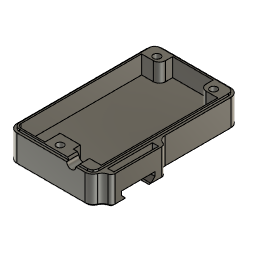
DisplayCaseBottom (Autodesk Fusion 360 design; units mm, degrees)
Autodesk Fusion 360 part; units mm, degrees
sketch "Skizze1" plane through (0, 0, 0) normal (0, 0, 1) x (1, 0, 0)
  line L0 (0, 0) -> (20.8, 0)
  line L1 (20.8, 0) -> (20.8, 72)
  line L2 (20.8, 72) -> (0, 72)
  line L3 (0, 72) -> (0, 0)
  dimension "d1" = 20.8
  dimension "d2" = 72
  constraint horizontal L0
  constraint vertical L1
  constraint horizontal L2
  constraint vertical L3
  constraint coincident L0.start L3.end
  measures "d1" distance of L0.start L0.end
  measures "d2" distance of L0.end L1.end
extrude "Extrusion1" add sketch "Skizze1" along normal blind 6
sketch "Skizze2" plane through (0, 0, 0) normal (-1, 0, 0) x (0, -1, 0)
  line L0 (-72, 0) -> (0, 0)
  line L1 (0, 0) -> (0, 6)
  line L2 (0, 6) -> (-72, 6)
  line L3 (-72, 6) -> (-72, 0)
  line L4 (-24.5, 0) -> (-12, 0)
  line L5 (-12, 0) -> (-12, 1)
  line L6 (-12, 1) -> (-10, 3)
  line L7 (-10, 3) -> (-10, 5)
  line L8 (-10, 5) -> (-26.5, 5)
  line L9 (-26.5, 5) -> (-26.5, 3)
  line L10 (-26.5, 3) -> (-24.5, 1)
  line L11 (-24.5, 1) -> (-24.5, 0)
  dimension "d5" = 16.5
  dimension "d6" = 1
  dimension "d7" = 1
  dimension "d8" = 45
  dimension "d9" = 45
  dimension "d10" = 2
  dimension "d11" = 2
  dimension "d12" = 2
  dimension "d13" = 10
  constraint coincident L0 L4.start
  constraint coincident L0 L4.end
  constraint perpendicular L4 L5
  constraint perpendicular L4 L7
  constraint perpendicular L7 L8
  constraint perpendicular L8 L9
  constraint perpendicular L8 L11
  measures "d5" distance of L7.end L8.end
  measures "d6" distance of L4.start L10.end
  measures "d7" distance of L4.end L5.end
  measures "d8" angle of L5 L6
  measures "d9" angle of L10 L11
  measures "d10" vertical distance of L5.end L6.end
  measures "d11" distance of L6.end L7.end
  measures "d12" distance of L8.end L9.end
  measures "d13" horizontal distance of L0.end L7.end
extrude "Extrusion2" cut sketch "Skizze2" against normal through all contours L0 L4 L5 L6 L7 L8 L9 L10 L11
sketch "Skizze3" plane through (0, 0, 6) normal (0, 0, 1) x (-1, 0, 0)
  line L0 (0, -72) -> (0, 0)
  line L1 (0, 0) -> (-20.8, 0)
  line L2 (-20.8, 0) -> (-20.8, -72)
  line L3 (-20.8, -72) -> (0, -72)
  line L4 (0, -72) -> (-20.8, -72)
  line L5 (-20.8, -72) -> (-20.8, 0)
  line L6 (-20.8, 0) -> (0, 0)
  line L7 (0, 0) -> (0, -2)
  line L8 (0, -2) -> (-18.8, -2)
  line L9 (-18.8, -2) -> (-18.8, -70)
  line L10 (-18.8, -70) -> (0, -70)
  line L11 (0, -70) -> (0, -72)
  dimension "d15" = 2
  dimension "d16" = 2
  dimension "d17" = 2
  constraint coincident L0.start L3.end
  constraint coincident L2.end L3.start
  constraint coincident L1.end L2.start
  constraint coincident L0.end L1.start
  constraint coincident L0 L7.end
  constraint perpendicular L7 L8
  constraint perpendicular L8 L9
  constraint coincident L0 L10.end
  constraint perpendicular L0 L10
  measures "d15" distance of L0.start L10.end
  measures "d16" distance of L5 L9
  measures "d17" distance of L6 L8
extrude "Extrusion3" add sketch "Skizze3" along normal blind 8 contours L0 L1 L2 L3 L4 L5 L6 L7 L8 L9 L10 L11
sketch "Skizze4" plane through (0, 0, 14) normal (0, 0, 1) x (-1, 0, 0)
  line L0 (0, -70) -> (-18.8, -70)
  line L1 (-18.8, -70) -> (-18.8, -2)
  line L2 (-18.8, -2) -> (0, -2)
  line L3 (0, -70) -> (-18.8, -70)
  line L4 (-18.8, -70) -> (-18.8, -2)
  line L5 (-18.8, -2) -> (0, -2)
  line L6 (0, -2) -> (0, -1.2)
  line L7 (0, -1.2) -> (-19.6, -1.2)
  line L8 (-19.6, -1.2) -> (-19.6, -70.8)
  line L9 (-19.6, -70.8) -> (0, -70.8)
  line L10 (0, -70.8) -> (0, -70)
  dimension "d49" = 0.8
  dimension "d50" = 0.8
  dimension "d51" = 0.8
  constraint coincident L0.start L3.start
  constraint coincident L0.end L1.start
  constraint coincident L1.end L2.start
  constraint coincident L2.end L5.end
  constraint perpendicular L2 L6
  constraint perpendicular L6 L7
  constraint perpendicular L3 L8
  constraint perpendicular L8 L9
  constraint perpendicular L3 L10
  measures "d49" distance of L9.end L0.start
  measures "d50" distance of L0.end L8
  measures "d51" distance of L2.end L6.end
extrude "Extrusion4" add sketch "Skizze4" along normal blind 1
sketch "Skizze5" plane through (0, 0, 6) normal (0, 0, 1) x (-1, 0, 0)
  line L0 (0, -2) -> (-18.8, -2)
  line L1 (-18.8, -2) -> (-18.8, -70)
  line L2 (-18.8, -70) -> (0, -70)
  line L3 (0, -70) -> (0, -2)
  line L4 (-18.8, -70) -> (-10, -70)
  line L5 (-10, -70) -> (-10, -63.5)
  line L6 (-10, -63.5) -> (-18.8, -63.5)
  line L7 (-18.8, -63.5) -> (-18.8, -70)
  dimension "d25" = 10
  dimension "d26" = 6.5
  constraint horizontal L4
  constraint vertical L5
  constraint horizontal L6
  constraint vertical L7
  constraint coincident L1.end L2.start
  measures "d25" distance of L3 L5.end
  measures "d26" distance of L4.end L5.end
extrude "Extrusion5" add sketch "Skizze5" along normal blind 9 contours L1 L2 L4 L5 L6 L7
sketch "Skizze7" plane through (0, 0, 0) normal (0, 0, -1) x (1, 0, 0)
  line L0 (20.8, -24.5) -> (0, -24.5)
  line L1 (0, -24.5) -> (0, -72)
  line L2 (0, -72) -> (20.8, -72)
  line L3 (20.8, -72) -> (20.8, -24.5)
  point P0 (14, -66.25)
  dimension "d31" = 14
  dimension "d32" = 5.75
  measures "d31" horizontal distance of origin P0
  measures "d32" distance of L2 P0
hole "Bohrung1" at (14, 66.25, 0) direction (0, 0, 1) diameter 3.5 end through all counterbore diameter 6.5 counterbore depth 4
chamfer "Fase1" distance 1.5 angle 45 1 edges at (15.6316, 66.8828, 4)
sketch "Skizze8" plane through (0, 0, 6) normal (0, 0, 1) x (-1, 0, 0)
  line L0 (-18.8, -63.5) -> (-10, -63.5)
  line L1 (-10, -63.5) -> (-10, -70)
  line L2 (-10, -70) -> (0, -70)
  line L3 (0, -70) -> (0, -2)
  line L4 (0, -2) -> (-18.8, -2)
  line L5 (-18.8, -2) -> (-18.8, -63.5)
  line L6 (0, -2) -> (-5, -2)
  line L7 (-5, -2) -> (-5, -9.5)
  line L8 (-5, -9.5) -> (0, -9.5)
  line L9 (0, -9.5) -> (0, -2)
  dimension "d38" = 5
  dimension "d39" = 9.5
  constraint horizontal L6
  constraint vertical L7
  constraint horizontal L8
  constraint vertical L9
  constraint coincident L3.end L4.start
  measures "d38" distance of L3.end L6.end
  measures "d39" vertical distance of origin L7.end
extrude "Extrusion6" add sketch "Skizze8" along normal blind 9 contours L3 L4 L6 L7 L8 L9
sketch "Skizze9" plane through (0, 0, 0) normal (0, 0, -1) x (1, 0, 0)
  line L0 (0, -12) -> (20.8, -12)
  line L1 (20.8, -12) -> (20.8, 0)
  line L2 (20.8, 0) -> (0, 0)
  line L3 (0, 0) -> (0, -12)
  point P0 (0, -4.5)
  dimension "d42" = 4.5
  constraint coincident L3 P0
  measures "d42" distance of L2.end P0
hole "Bohrung2" at (0, 4.5, 0) direction (0, 0, 1) diameter 3.5 depth 16 tip angle 180 counterbore diameter 6.5 counterbore depth 6
chamfer "Fase2" distance 1.5 angle 45 1 edges at (1.75, 4.5, 6)
fillet "Abrundung6" radius 2 1 edges at (18.8, 2, 10.5)
fillet "Abrundung2" radius 2.8 2 edges at (19.6, 1.2, 14.5) (19.6, 70.8, 14.5)
fillet "Abrundung4" radius 4 2 edges at (20.8, 0, 7) (20.8, 72, 7)
fillet "Abrundung5" radius 3 1 edges at (10, 63.5, 10.5)
mirror "Spiegeln1" about plane through (0, 0, 0) normal (1, 0, 0) of bodies 1 merged
sketch "Skizze11" plane through (0, 0, 6) normal (0, 0, 1) x (-1, 0, 0)
  line L0 (-18.8, -4) -> (-18.8, -63.5)
  line L1 (-18.8, -63.5) -> (-13, -63.5)
  arc A0 (-10, -66.5) -> (-13, -63.5) centre (-13, -66.5) ccw
  line L2 (-10, -66.5) -> (-10, -70)
  line L3 (-10, -70) -> (10, -70)
  line L4 (10, -70) -> (10, -66.5)
  arc A1 (13, -63.5) -> (10, -66.5) centre (13, -66.5) ccw
  line L5 (13, -63.5) -> (18.8, -63.5)
  line L6 (18.8, -63.5) -> (18.8, -4)
  line L7 (16.8, -2) -> (5, -2)
  line L8 (5, -2) -> (5, -9.5)
  line L9 (5, -9.5) -> (-5, -9.5)
  line L10 (-5, -9.5) -> (-5, -2)
  line L11 (-5, -2) -> (-16.8, -2)
  line L12 (-5, -2) -> (-18.8, -2)
  line L13 (-18.8, -2) -> (-18.8, -6)
  line L14 (-18.8, -6) -> (-5, -6)
  line L15 (-5, -6) -> (-5, -2)
  arc A2 (-16.8, -2) -> (-18.8, -4) centre (-16.8, -4) ccw
  arc A3 (18.8, -4) -> (16.8, -2) centre (16.8, -4) ccw
  dimension "d68" = 4
  constraint horizontal L12
  constraint vertical L13
  constraint horizontal L14
  constraint vertical L15
  constraint coincident L0 L13.end
  constraint coincident L10.end L11.start
  measures "d68" distance of L12.end L13.end
extrude "Extrusion7" add sketch "Skizze11" along normal blind 9 contours L0 L10 L11 L12 L13 L14 L15 A2 | L12 L13 A2
sketch "Skizze10" plane through (0, 0, 0) normal (0, -1, 0) x (1, 0, 0)
  line L0 (16.8, 0) -> (16.8, 14)
  line L1 (16.8, 14) -> (-16.8, 14)
  line L2 (-16.8, 14) -> (-16.8, 0)
  circle A0 centre (10, 14) radius 2.25
  line L3 (-16.8, 0) -> (16.8, 0)
  dimension "d66" = 4.5
  dimension "d67" = 10
  constraint coincident L1 A0.centre
  measures "d66" diameter of A0
  measures "d67" horizontal distance of origin A0.centre
extrude "Extrusion8" cut sketch "Skizze10" against normal blind 12 contours L1 A0 | L1 A0
chamfer "Fase5" distance 1 angle 45 3 edges at (7.9844, 3.6, 15) (12.0156, 3.6, 15) (7.9844, 3.6, 15)
sketch "Skizze16" plane through (20.8, 0, 0) normal (1, 0, 0) x (0, 1, 0)
  line L0 (68, 0) -> (68, 14)
  line L1 (68, 14) -> (4, 14)
  line L2 (4, 14) -> (4, 0)
  line L3 (4, 0) -> (12, 0)
  line L4 (12, 0) -> (12, 1)
  line L5 (12, 1) -> (10, 3)
  line L6 (10, 3) -> (10, 5)
  line L7 (10, 5) -> (26.5, 5)
  line L8 (26.5, 5) -> (26.5, 3)
  line L9 (26.5, 3) -> (24.5, 1)
  line L10 (24.5, 1) -> (24.5, 0)
  line L11 (24.5, 0) -> (68, 0)
  line L12 (5, 14) -> (31.5, 14)
  line L13 (31.5, 14) -> (31.5, 0)
  line L14 (31.5, 0) -> (5, 0)
  line L15 (5, 0) -> (5, 14)
  dimension "d100" = 5
  dimension "d101" = 5
  constraint horizontal L12
  constraint vertical L13
  constraint horizontal L14
  constraint vertical L15
  constraint coincident L11 L13.end
  constraint coincident L1 L12.start
  measures "d100" horizontal distance of L7.end L13.end
  measures "d101" distance of L6.end L15
extrude "Extrusion12" add sketch "Skizze16" along normal blind 4 contours L1 L3 L4 L5 L6 L7 L8 L9 L10 L11 L12 L13 L14 L15
sketch "Skizze17" plane through (0, 0, 14) normal (0, 0, 1) x (-1, 0, 0)
  line L0 (-12.25, -1.2) -> (-12.25, 0)
  line L1 (-12.25, 0) -> (-16.8, 0)
  arc A0 (-16.8, 0) -> (-20.8, -4) centre (-16.8, -4) ccw
  line L2 (-20.8, -4) -> (-20.8, -5)
  line L3 (-20.8, -5) -> (-24.8, -5)
  line L4 (-24.8, -5) -> (-24.8, -31.5)
  line L5 (-24.8, -31.5) -> (-20.8, -31.5)
  line L6 (-20.8, -31.5) -> (-20.8, -68)
  arc A1 (-20.8, -68) -> (-16.8, -72) centre (-16.8, -68) ccw
  line L7 (-16.8, -72) -> (16.8, -72)
  arc A2 (16.8, -72) -> (20.8, -68) centre (16.8, -68) ccw
  line L8 (20.8, -68) -> (20.8, -4)
  arc A3 (20.8, -4) -> (16.8, 0) centre (16.8, -4) ccw
  line L9 (16.8, 0) -> (-7.75, 0)
  line L10 (-7.75, 0) -> (-7.75, -1.2)
  line L11 (-7.75, -1.2) -> (16.8, -1.2)
  arc A4 (19.6, -4) -> (16.8, -1.2) centre (16.8, -4) ccw
  line L12 (19.6, -4) -> (19.6, -68)
  arc A5 (16.8, -70.8) -> (19.6, -68) centre (16.8, -68) ccw
  line L13 (16.8, -70.8) -> (-16.8, -70.8)
  arc A6 (-19.6, -68) -> (-16.8, -70.8) centre (-16.8, -68) ccw
  line L14 (-19.6, -68) -> (-19.6, -4)
  arc A7 (-18.8, -2.0404) -> (-19.6, -4) centre (-16.8, -4) ccw
  line L15 (-18.8, -2.0404) -> (-18.8, -2)
  line L16 (-18.8, -2) -> (-18.7596, -2)
  arc A8 (-16.8, -1.2) -> (-18.7596, -2) centre (-16.8, -4) ccw
  line L17 (-16.8, -1.2) -> (-12.25, -1.2)
  line L18 (-20.8, -29.25) -> (-23.8, -29.25)
  line L19 (-23.8, -29.25) -> (-23.8, -7.25)
  line L20 (-23.8, -7.25) -> (-20.8, -7.25)
  line L21 (-20.8, -7.25) -> (-20.8, -29.25)
  dimension "d104" = 1
  dimension "d105" = 22
  dimension "d106" = 2.25
  dimension "d107" = 2.25
  dimension "d108" = 3
  constraint horizontal L18
  constraint vertical L19
  constraint horizontal L20
  constraint vertical L21
  measures "d104" horizontal distance of L3.end L19.end
  measures "d105" distance of L18.end L19.end
  measures "d106" distance of L3 L19.end
  measures "d107" vertical distance of L4.end L18.end
  measures "d108" distance of L19.end L20.end
extrude "Extrusion13" cut sketch "Skizze17" against normal blind 7 contours L18 L19 L20 L21
fillet "Abrundung11" radius 4 2 edges at (20.8, 5, 7) (20.8, 31.5, 7)
fillet "Abrundung12" radius 2 2 edges at (24.8, 5, 7) (24.8, 31.5, 7)
chamfer "Fase7" distance 1 angle 45 15 edges at (19.0361, 0.6834, 0) (21.6018, 4.0273, 0) (24.3723, 5.5944, 0) (24.8, 9.4152, 0) (-20.8, 8, 0) (-19.6284, 1.1716, 0) (0, 0, 0) (20.8, 51.75, 0) (19.6284, 70.8284, 0) (0, 72, 0) (-19.6284, 70.8284, 0) (-20.8, 46.25, 0) (24.8, 27.1716, 0) (24.433, 30.9978, 0) (21.534, 33.1906, 0)
equation "d1 = ( 41.6 / 2 ) * 1 mm"
equation "d106 = d107"
